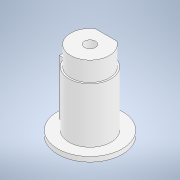
# Autodesk Inventor part: wheel_adapt
Saved by Autodesk Inventor 2020.4 (Build 244396000, 396)
## iProperties
Created: 2020-06-12
Part Number: wheel_adapt
Material: Generic
Document SubType Name: Modeling
Designer: Tarsoly
Density: 1 g/cm^3
Appearance: Default
Author: Tarsoly
Autodesk Inventor part; units mm, degrees
ref_plane "YZ Plane" through (0, 0, 0) normal (1, 0, 0) x (0, 1, 0)
ref_plane "XZ Plane" through (0, 0, 0) normal (0, 1, 0) x (-1, 0, 0)
ref_plane "XY Plane" through (0, 0, 0) normal (0, 0, 1) x (1, 0, 0)
sketch "Sketch1" plane through (0, 0, 0) normal (0, 1, 0) x (-1, 0, 0)
  circle A0 centre (0, 0) radius 6.5
  line L0 (7.76, 1.75) -> (6.26, 1.75)
  line L1 (6.26, 1.75) -> (6.26, -1.75)
  line L2 (6.26, -1.75) -> (7.76, -1.75)
  line L3 (7.76, -1.75) -> (7.76, 1.75)
  dimension "d0" = 13
  dimension "d8" = 1.5
  dimension "d9" = 3.5
  constraints: 8 end point, 2 parallel, 2 point on circle, 1 centre point, 1 coincident, 1 horizontal, 1 perpendicular
  measures "d0" diameter of A0
  measures "d8" distance of L2.end L1.end
  measures "d9" distance of L1.end L0.end
extrude "Extrusion1" add sketch "Sketch1" along normal blind 17
sketch "Sketch2" plane through (0, 0, 0) normal (0, -1, 0) x (0, 0, -1)
  circle A0 centre (0, 0) radius 10
  dimension "d3" = 20
  constraints: 1 centre point, 1 coincident
  measures "d3" diameter of A0
extrude "Extrusion2" add sketch "Sketch2" along normal blind 1.5
sketch "Sketch4" plane through (0, 17, 0) normal (0, 1, 0) x (1, 0, 0)
  circle A0 centre (0, 0) radius 6
  arc A1 (-6.26, -1.75) -> (-6.26, 1.75) centre (0, 0) ccw projected
  line L0 (4.1533, 5) -> (-4.1533, 5)
  point P0 (3.3166, 5)
  point P1 (-3.3166, 5)
  dimension "d10" = 12
  dimension "d27" = 5
  constraints: 2 end point, 2 point on circle, 1 centre point, 1 coincident, 1 horizontal
  measures "d10" diameter of A0
  measures "d27" distance from line of L0 point (0, 0)
extrude "Extrusion3" add sketch "Sketch4" along normal blind 6 contours A0 L0 picked at (-0.7721, -1.8319)
sketch "Sketch5" plane through (0, 23, 0) normal (0, 1, 0) x (1, 0, 0)
  point P0 (0, 0)
  point P1 (0, 0)
  constraints: 1 coincident
hole "Hole1" at (0, 23, 0) direction (0, -1, 0) diameter 3.4 depth 9 tip angle 118 clearance for "Hex Head Cap Screw ISO 24017" size "M3" standard "ISO"
sketch "Sketch6" plane through (0, 0, 0) normal (0, 0, 1) x (1, 0, 0)
  circle A0 centre (0, 20) radius 0.75
  line L0 (6, 23) -> (-6, 23) projected
  line L1 (0, -4.6) -> (0, 27.6) projected
  point P0 (0, 0)
  dimension "d21" = 1.5
  dimension "d26" = 3
  constraints: 1 centre point, 1 point on line
  measures "d21" diameter of A0
  measures "d26" distance from line of L0 A0.centre
extrude "Extrusion4" cut sketch "Sketch6" against normal up to surface round surface about axis through (0, 17, 0) along (0, 1, 0) radius 6 far side no
body "Solid1"
